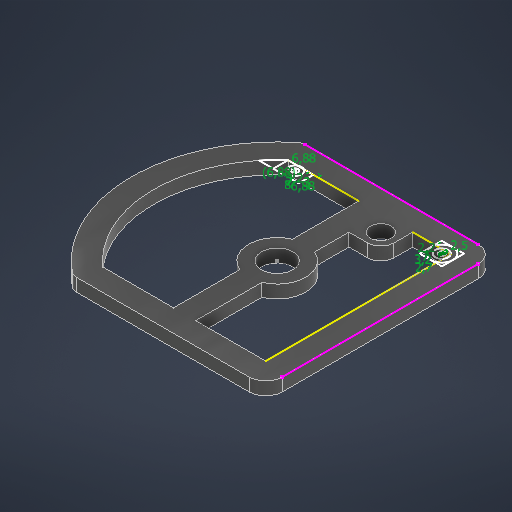
# Autodesk Inventor part: Acrílicos superiores
Saved by Autodesk Inventor 2026.2 (Build 302298000, 298)
## iProperties
Created: 2026-02-09
Part Number: Acrílicos superiores
Material: Generic
Document SubType Name: Modeling
Designer: 06aar
Density: 1 g/cm^3
Appearance: Dark Gray
Author: 06aar
Autodesk Inventor part; units mm, degrees
ref_plane "YZ Plane" through (0, 0, 0) normal (1, 0, 0) x (0, 1, 0)
ref_plane "XZ Plane" through (0, 0, 0) normal (0, 1, 0) x (-1, 0, 0)
ref_plane "XY Plane" through (0, 0, 0) normal (0, 0, 1) x (1, 0, 0)
sketch "Sketch1" plane through (0, 0, 0) normal (0, 1, 0) x (-1, 0, 0)
  line L0 (46.9204, 62.223) -> (-47, 62.223)
  line L1 (-47, -62.223) -> (46.9204, -62.223)
  line L2 (-56, 53.223) -> (-56, -53.223)
  arc A0 (50.0907, -61.0894) -> (50.0907, 61.0894) centre (0, 0) ccw
  arc A1 (50.0907, 61.0894) -> (46.9204, 62.223) centre (46.9204, 57.223) ccw
  arc A2 (46.9204, -62.223) -> (50.0907, -61.0894) centre (46.9204, -57.223) ccw
  arc A3 (-47, 62.223) -> (-56, 53.223) centre (-47, 53.223) ccw
  arc A4 (-56, -53.223) -> (-47, -62.223) centre (-47, -53.223) ccw
  line L3 (-44, 50.223) -> (44.3469, 50.223)
  arc A5 (44.3469, -50.223) -> (44.3469, 50.223) centre (0, 0) ccw
  line L4 (44.3469, -50.223) -> (-44, -50.223)
  line L5 (-44, -50.223) -> (-44, 50.223)
  circle A6 centre (0, 0) radius 8.5
  circle A7 centre (0, 0) radius 15.5
  line L6 (-6, -14.2916) -> (-6, -50.223)
  line L7 (0, 0) -> (0, -8.5)
  line L8 (6, -14.2916) -> (6, -50.223)
  line L9 (0, 0) -> (8.5, 0)
  line L10 (-6, 14.2916) -> (-6, 50.223)
  line L11 (6, 14.2916) -> (6, 50.223)
  circle A8 centre (-14.65, -41.573) radius 5.65
  line L12 (-14.65, -41.573) -> (-14.65, -50.223)
  line L13 (-6, -41.573) -> (-14.65, -41.573)
  line L14 (-6, -32.923) -> (-16.15, -32.923)
  line L15 (-23.3, -40.073) -> (-23.3, -50.223)
  arc A9 (-16.15, -32.923) -> (-23.3, -40.073) centre (-16.15, -40.073) ccw
  point P0 (48.6754, 62.223)
  point P1 (48.6754, -62.223)
  point P2 (-23.3, -50.223)
  point P3 (-44, -32.923)
  dimension "d2" = 62.223
  dimension "d4" = 56
  dimension "d5" = 62.223
  dimension "d6" = 79
  dimension "d7" = 5
  dimension "d8" = 9
  dimension "d18" = 12
  dimension "d21" = 17
  dimension "d22" = 7
  dimension "d24" = 6
  dimension "d41" = 11.3
  dimension "d45" = 8.65
  dimension "d46" = 8.65
  dimension "d47" = 17.3
  dimension "d48" = 3
  dimension "d49" = 90
  dimension "d50" = 7.15
  constraints: 32 end point, 18 point on circle, 10 tangent, 9 centre point, 9 point on line, 6 symmetric about line, 4 horizontal, 3 coincident, 2 equal radius, 2 parallel, 2 perpendicular, 2 vertical, 6 other
  measures "d2" distance from line of point (0, 0) L0
  measures "d4" distance from line of L2 point (0, 0)
  measures "d5" distance from line of point (0, 0) L1
  measures "d6" radius of A0
  measures "d7" radius of A1
  measures "d8" radius of A3
  measures "d18" distance between parallel lines of L0 L3
  measures "d21" diameter of A6
  measures "d24" distance from line of L7.end L6
  measures "d41" diameter of A8
  measures "d45" distance of L12.start L12.end
  measures "d46" distance of L13.start L12.start
  measures "d47" distance between parallel lines of L4 L14
  measures "d48" distance edge to line of A8 L15
  measures "d49" angle of L4 L15
  measures "d50" radius of A9
extrude "Extrusion1" add sketch "Sketch1" against normal blind 7 contours A1 A0 A2 L1 A4 L2 A3 L0 | L3 L11 A7 L10 | A7 | L15 A9 L14 L6 L13 A8 L12 L4 | A7 L8 L4 L6 | L12 A8 L13 L6 L4
sketch "Sketch4" plane through (0, 0, 0) normal (0, 1, 0) x (1, 0, 0)
  circle A0 centre (-37.4674, 47.2232) radius 1.6
  circle A1 centre (41.3, 48.0232) radius 1.6
  line L0 (-44.3469, 50.223) -> (-6, 50.223) projected
  circle A2 centre (-37.4674, 47.2232) radius 3.5
  line L1 (-30.5874, 42.223) -> (-44.3469, 42.223)
  line L2 (-44.3469, 42.223) -> (-44.3469, 50.223)
  line L3 (-44.3469, 50.223) -> (-30.5874, 50.223)
  line L4 (-30.5874, 50.223) -> (-30.5874, 42.223)
  line L5 (-44.3469, 42.223) -> (-52.0213, 42.223)
  arc A3 (-44.3469, 50.223) -> (-52.0213, 42.223) centre (0, 0) ccw
  line L6 (44, 50.223) -> (44, -50.223) projected
  line L7 (23.3, 50.223) -> (44, 50.223) projected
  circle A4 centre (41.3, 48.0232) radius 3.5
  line L8 (47, 62.223) -> (-46.9204, 62.223) projected
  line L9 (56, -53.223) -> (56, 53.223) projected
  circle A5 centre (41.3, 48.0232) radius 6
  line L10 (35.3, 42.0232) -> (47.3, 42.0232)
  line L11 (47.3, 42.0232) -> (47.3, 54.0232)
  line L12 (47.3, 54.0232) -> (35.3, 54.0232)
  line L13 (35.3, 54.0232) -> (35.3, 42.0232)
  point P0 (35.3, 50.223)
  point P1 (44, 42.0232)
  point P2 (-39.2706, 50.223)
  point P3 (-35.6642, 50.223)
  dimension "d61" = 2.9998
  dimension "d62" = 6.8795
  dimension "d63" = 3.2
  dimension "d64" = 7
  dimension "d65" = 6.8795
  dimension "d66" = 6.88
  dimension "d67" = 8
  dimension "d68" = 3.2
  dimension "d69" = 2.7
  dimension "d70" = 2.1998
  dimension "d71" = 7
  dimension "d77" = 2.5
  constraints: 18 end point, 6 centre point, 4 coincident, 4 parallel, 4 tangent, 3 horizontal, 2 perpendicular, 2 point on circle
  measures "d61" distance from line of L0 A0.centre
  measures "d62" horizontal distance of L0.start A0.centre
  measures "d63" diameter of A0
  measures "d64" diameter of A2
  measures "d65" distance from line of A0.centre L2
  measures "d66" distance from line of L4 A0.centre
  measures "d67" distance between parallel lines of L0 L1
  measures "d68" diameter of A1
  measures "d69" distance from line of L6 A1.centre
  measures "d70" distance from line of L7 A1.centre
  measures "d71" diameter of A4
  measures "d77" radial gap between concentric circles of A4 A5
body "Solid1"
